Autodesk Fusion 360 part; units mm, degrees
note: some values were not read from the file. Set by a fixed rule: which sketch regions a step uses.
(part 14 of 20)
  spline S78 degree 5 poles (15.0758, 27.0873) (15.0737, 27.0855) (15.0696, 27.082) (15.0635, 27.0767) (15.0553, 27.0697) (15.045, 27.061) (15.0349, 27.0522) (15.0247, 27.0435) (15.0146, 27.0347) (15.0045, 27.026) (14.9945, 27.0173) (14.9845, 27.0086) (14.9745, 26.9999) (14.9646, 26.9912) (14.9547, 26.9825) (14.9448, 26.9738) (14.935, 26.9651) (14.9252, 26.9565) (14.9154, 26.9478) (14.9057, 26.9392) (14.896, 26.9305) (14.8863, 26.9219) (14.8767, 26.9133) (14.8671, 26.9047) (14.8576, 26.8961) (14.8481, 26.8875) (14.8386, 26.8789) (14.8291, 26.8703) (14.8197, 26.8618) (14.8104, 26.8532) (14.801, 26.8447) (14.7917, 26.8361) (14.7824, 26.8276) (14.7732, 26.8191) (14.764, 26.8106) (14.7549, 26.8021) (14.7457, 26.7937) (14.7366, 26.7852) (14.7276, 26.7767) (14.7186, 26.7683) (14.7096, 26.7599) (14.7006, 26.7515) (14.6917, 26.7431) (14.6829, 26.7347) (14.674, 26.7263) (14.6652, 26.7179) (14.6565, 26.7096) (14.6477, 26.7012) (14.639, 26.6929) (14.6304, 26.6846) (14.6218, 26.6763) (14.6132, 26.668) (14.6046, 26.6597) (14.5961, 26.6514) (14.5877, 26.6432) (14.5792, 26.635) (14.5708, 26.6267) (14.5625, 26.6185) (14.5541, 26.6103) (14.5459, 26.6022) (14.5376, 26.594) (14.5294, 26.5858) (14.5212, 26.5777) (14.5131, 26.5696) (14.505, 26.5615) (14.4969, 26.5534) (14.4889, 26.5453) (14.4809, 26.5373) (14.4729, 26.5292) (14.465, 26.5212) (14.4571, 26.5132) (14.4493, 26.5052) (14.4415, 26.4972) (14.4337, 26.4893) (14.426, 26.4813) (14.4183, 26.4734) (14.4106, 26.4655) (14.403, 26.4576) (14.3954, 26.4497) (14.3879, 26.4419) (14.3804, 26.434) (14.3729, 26.4262) (14.3655, 26.4184) (14.3581, 26.4106) (14.3508, 26.4029) (14.3435, 26.3951) (14.3362, 26.3874) (14.3289, 26.3797) (14.3217, 26.372) (14.3146, 26.3643) (14.3075, 26.3567) (14.3004, 26.3491) (14.2933, 26.3414) (14.2863, 26.3339) (14.2794, 26.3263) (14.2724, 26.3188) (14.2656, 26.3112) (14.2587, 26.3037) (14.2519, 26.2962) (14.2451, 26.2888) (14.2384, 26.2813) (14.2317, 26.2739) (14.225, 26.2665) (14.2184, 26.2592) (14.2119, 26.2518) (14.2053, 26.2445) (14.1988, 26.2372) (14.1924, 26.2299) (14.1859, 26.2227) (14.1796, 26.2154) (14.1732, 26.2082) (14.1669, 26.201) (14.1607, 26.1939) (14.1544, 26.1868) (14.1483, 26.1796) (14.1421, 26.1726) (14.136, 26.1655) (14.13, 26.1585) (14.1239, 26.1515) (14.118, 26.1445) (14.112, 26.1375) (14.1061, 26.1306) (14.1003, 26.1237) (14.0945, 26.1168) (14.0887, 26.11) (14.0829, 26.1032) (14.0772, 26.0964) (14.0716, 26.0896) (14.066, 26.0829) (14.0604, 26.0762) (14.0549, 26.0695) (14.0494, 26.0629) (14.0439, 26.0563) (14.0385, 26.0497) (14.0332, 26.0431) (14.0278, 26.0366) (14.0225, 26.0301) (14.0173, 26.0236) (14.0121, 26.0172) (14.0069, 26.0108) (14.0018, 26.0044) (13.9967, 25.9981) (13.9917, 25.9918) (13.9867, 25.9855) (13.9818, 25.9793) (13.9769, 25.9731) (13.972, 25.9669) (13.9672, 25.9608) (13.9624, 25.9547) (13.9576, 25.9486) (13.9529, 25.9426) (13.9483, 25.9366) (13.9437, 25.9306) (13.9391, 25.9247) (13.9346, 25.9188) (13.9301, 25.913) (13.9257, 25.9072) (13.9213, 25.9014) (13.9169, 25.8957) (13.9126, 25.89) (13.9083, 25.8843) (13.9041, 25.8787) (13.8999, 25.8731) (13.8958, 25.8676) (13.8917, 25.8621) (13.8876, 25.8566) (13.8836, 25.8512) (13.8797, 25.8458) (13.8758, 25.8405) (13.8719, 25.8352) (13.8681, 25.8299) (13.8643, 25.8247) (13.8605, 25.8195) (13.8568, 25.8144) (13.8532, 25.8093) (13.8496, 25.8043) (13.846, 25.7993) (13.8425, 25.7944) (13.839, 25.7895) (13.8356, 25.7847) (13.8322, 25.7799) (13.8289, 25.7751) (13.8256, 25.7704) (13.8224, 25.7658) (13.8192, 25.7612) (13.816, 25.7566) (13.8129, 25.7521) (13.8098, 25.7476) (13.8068, 25.7432) (13.8039, 25.7389) (13.8009, 25.7346) (13.7981, 25.7304) (13.7952, 25.7262) (13.7925, 25.722) (13.7897, 25.718) (13.787, 25.7139) (13.7844, 25.71) (13.7818, 25.706) (13.7793, 25.7022) (13.7768, 25.6984) (13.7743, 25.6947) (13.7719, 25.691) (13.7696, 25.6874) (13.7673, 25.6838) (13.765, 25.6803) (13.7628, 25.6769) (13.7607, 25.6735) (13.7586, 25.6702) (13.7565, 25.667) (13.7545, 25.6638) (13.7526, 25.6607) (13.7506, 25.6577) (13.7488, 25.6547) (13.747, 25.6518) (13.7452, 25.6489) (13.7435, 25.6462) (13.7419, 25.6435) (13.7403, 25.6409) (13.7387, 25.6383) (13.7372, 25.6358) (13.7358, 25.6334) (13.7344, 25.6311) (13.733, 25.6289) (13.7317, 25.6267) (13.7305, 25.6246) (13.7293, 25.6226) (13.7282, 25.6207) (13.7271, 25.6188) (13.7261, 25.6171) (13.7251, 25.6154) (13.7242, 25.6138) (13.7233, 25.6123) (13.7225, 25.6109) (13.7217, 25.6096) (13.721, 25.6083) (13.7204, 25.6072) (13.7198, 25.6061) (13.7193, 25.6052) (13.7188, 25.6043) (13.7184, 25.6036) (13.718, 25.6029) (13.7178, 25.6025) (13.7176, 25.6022) (13.7175, 25.602) (13.7175, 25.6019) knots -1 -1 -1 -1 -1 -1 -0.99583333 -0.99166667 -0.9875 -0.98333333 -0.97916667 -0.975 -0.97083333 -0.96666667 -0.9625 -0.95833333 -0.95416667 -0.95 -0.94583333 -0.94166667 -0.9375 -0.93333333 -0.92916667 -0.925 -0.92083333 -0.91666667 -0.9125 -0.90833333 -0.90416667 -0.9 -0.89583333 -0.89166667 -0.8875 -0.88333333 -0.87916667 -0.875 -0.87083333 -0.86666667 -0.8625 -0.85833333 -0.85416667 -0.85 -0.84583333 -0.84166667 -0.8375 -0.83333333 -0.82916667 -0.825 -0.82083333 -0.81666667 -0.8125 -0.80833333 -0.80416667 -0.8 -0.79583333 -0.79166667 -0.7875 -0.78333333 -0.77916667 -0.775 -0.77083333 -0.76666667 -0.7625 -0.75833333 -0.75416667 -0.75 -0.74583333 -0.74166667 -0.7375 -0.73333333 -0.72916667 -0.725 -0.72083333 -0.71666667 -0.7125 -0.70833333 -0.70416667 -0.7 -0.69583333 -0.69166667 -0.6875 -0.68333333 -0.67916667 -0.675 -0.67083333 -0.66666667 -0.6625 -0.65833333 -0.65416667 -0.65 -0.64583333 -0.64166667 -0.6375 -0.63333333 -0.62916667 -0.625 -0.62083333 -0.61666667 -0.6125 -0.60833333 -0.60416667 -0.6 -0.59583333 -0.59166667 -0.5875 -0.58333333 -0.57916667 -0.575 -0.57083333 -0.56666667 -0.5625 -0.55833333 -0.55416667 -0.55 -0.54583333 -0.54166667 -0.5375 -0.53333333 -0.52916667 -0.525 -0.52083333 -0.51666667 -0.5125 -0.50833333 -0.50416667 -0.5 -0.49583333 -0.49166667 -0.4875 -0.48333333 -0.47916667 -0.475 -0.47083333 -0.46666667 -0.4625 -0.45833333 -0.45416667 -0.45 -0.44583333 -0.44166667 -0.4375 -0.43333333 -0.42916667 -0.425 -0.42083333 -0.41666667 -0.4125 -0.40833333 -0.40416667 -0.4 -0.39583333 -0.39166667 -0.3875 -0.38333333 -0.37916667 -0.375 -0.37083333 -0.36666667 -0.3625 -0.35833333 -0.35416667 -0.35 -0.34583333 -0.34166667 -0.3375 -0.33333333 -0.32916667 -0.325 -0.32083333 -0.31666667 -0.3125 -0.30833333 -0.30416667 -0.3 -0.29583333 -0.29166667 -0.2875 -0.28333333 -0.27916667 -0.275 -0.27083333 -0.26666667 -0.2625 -0.25833333 -0.25416667 -0.25 -0.24583333 -0.24166667 -0.2375 -0.23333333 -0.22916667 -0.225 -0.22083333 -0.21666667 -0.2125 -0.20833333 -0.20416667 -0.2 -0.19583333 -0.19166667 -0.1875 -0.18333333 -0.17916667 -0.175 -0.17083333 -0.16666667 -0.1625 -0.15833333 -0.15416667 -0.15 -0.14583333 -0.14166667 -0.1375 -0.13333333 -0.12916667 -0.125 -0.12083333 -0.11666667 -0.1125 -0.10833333 -0.10416667 -0.1 -0.09583333 -0.09166667 -0.0875 -0.08333333 -0.07916667 -0.075 -0.07083333 -0.06666667 -0.0625 -0.05833333 -0.05416667 -0.05 -0.04583333 -0.04166667 -0.0375 -0.03333333 -0.02916667 -0.025 -0.02083333 -0.01666667 -0.0125 -0.00833333 -0.00416667 0 0 0 0 0 0
  line L164 (-13.578, 25.3417) -> (-13.7171, 25.6012)
  line L165 (-12.6495, 26.1461) -> (-12.6491, 26.1453)
  spline S79 degree 5 poles (17.8246, 25.363) (17.8224, 25.3615) (17.8179, 25.3584) (17.8112, 25.3539) (17.8023, 25.3477) (17.7913, 25.3401) (17.7802, 25.3325) (17.7692, 25.3248) (17.7583, 25.3172) (17.7473, 25.3096) (17.7364, 25.3019) (17.7256, 25.2943) (17.7147, 25.2867) (17.7039, 25.2791) (17.6932, 25.2715) (17.6825, 25.2639) (17.6718, 25.2563) (17.6611, 25.2487) (17.6505, 25.2411) (17.6399, 25.2335) (17.6294, 25.2259) (17.6189, 25.2184) (17.6084, 25.2108) (17.598, 25.2032) (17.5876, 25.1957) (17.5772, 25.1881) (17.5669, 25.1806) (17.5566, 25.1731) (17.5464, 25.1655) (17.5361, 25.158) (17.526, 25.1505) (17.5158, 25.143) (17.5057, 25.1355) (17.4956, 25.128) (17.4856, 25.1205) (17.4756, 25.113) (17.4657, 25.1055) (17.4557, 25.0981) (17.4458, 25.0906) (17.436, 25.0832) (17.4262, 25.0757) (17.4164, 25.0683) (17.4067, 25.0609) (17.397, 25.0534) (17.3873, 25.046) (17.3777, 25.0386) (17.3681, 25.0312) (17.3585, 25.0238) (17.349, 25.0165) (17.3395, 25.0091) (17.3301, 25.0017) (17.3207, 24.9944) (17.3113, 24.9871) (17.302, 24.9797) (17.2927, 24.9724) (17.2835, 24.9651) (17.2743, 24.9578) (17.2651, 24.9505) (17.2559, 24.9432) (17.2469, 24.936) (17.2378, 24.9287) (17.2288, 24.9215) (17.2198, 24.9142) (17.2108, 24.907) (17.2019, 24.8998) (17.1931, 24.8926) (17.1842, 24.8854) (17.1754, 24.8782) (17.1667, 24.8711) (17.158, 24.8639) (17.1493, 24.8568) (17.1407, 24.8496) (17.1321, 24.8425) (17.1235, 24.8354) (17.115, 24.8283) (17.1065, 24.8212) (17.0981, 24.8142) (17.0897, 24.8071) (17.0813, 24.8001) (17.073, 24.7931) (17.0647, 24.7861) (17.0565, 24.7791) (17.0483, 24.7721) (17.0401, 24.7651) (17.032, 24.7582) (17.0239, 24.7512) (17.0159, 24.7443) (17.0079, 24.7374) (16.9999, 24.7305) (16.992, 24.7236) (16.9841, 24.7168) (16.9763, 24.7099) (16.9685, 24.7031) (16.9607, 24.6963) (16.953, 24.6895) (16.9453, 24.6827) (16.9377, 24.6759) (16.9301, 24.6692) (16.9225, 24.6625) (16.915, 24.6558) (16.9075, 24.6491) (16.9001, 24.6424) (16.8927, 24.6357) (16.8854, 24.6291) (16.8781, 24.6225) (16.8708, 24.6159) (16.8636, 24.6093) (16.8564, 24.6027) (16.8492, 24.5962) (16.8421, 24.5897) (16.8351, 24.5831) (16.8281, 24.5767) (16.8211, 24.5702) (16.8142, 24.5638) (16.8073, 24.5573) (16.8004, 24.5509) (16.7936, 24.5446) (16.7869, 24.5382) (16.7801, 24.5319) (16.7735, 24.5255) (16.7668, 24.5192) (16.7602, 24.513) (16.7537, 24.5067) (16.7472, 24.5005) (16.7407, 24.4943) (16.7343, 24.4881) (16.7279, 24.482) (16.7216, 24.4758) (16.7153, 24.4697) (16.7091, 24.4636) (16.7029, 24.4576) (16.6967, 24.4515) (16.6906, 24.4455) (16.6845, 24.4395) (16.6785, 24.4336) (16.6725, 24.4277) (16.6666, 24.4218) (16.6607, 24.4159) (16.6549, 24.41) (16.6491, 24.4042) (16.6433, 24.3984) (16.6376, 24.3926) (16.6319, 24.3869) (16.6263, 24.3812) (16.6207, 24.3755) (16.6152, 24.3698) (16.6097, 24.3642) (16.6043, 24.3586) (16.5989, 24.353) (16.5935, 24.3475) (16.5882, 24.342) (16.583, 24.3365) (16.5778, 24.3311) (16.5726, 24.3257) (16.5675, 24.3203) (16.5624, 24.3149) (16.5574, 24.3096) (16.5524, 24.3043) (16.5475, 24.2991) (16.5426, 24.2939) (16.5378, 24.2887) (16.533, 24.2835) (16.5282, 24.2784) (16.5236, 24.2733) (16.5189, 24.2683) (16.5143, 24.2633) (16.5098, 24.2583) (16.5053, 24.2534) (16.5008, 24.2485) (16.4964, 24.2436) (16.492, 24.2388) (16.4877, 24.234) (16.4835, 24.2293) (16.4793, 24.2246) (16.4751, 24.2199) (16.471, 24.2153) (16.4669, 24.2107) (16.4629, 24.2062) (16.459, 24.2017) (16.455, 24.1972) (16.4512, 24.1928) (16.4474, 24.1884) (16.4436, 24.1841) (16.4399, 24.1798) (16.4362, 24.1755) (16.4326, 24.1713) (16.4291, 24.1672) (16.4256, 24.1631) (16.4221, 24.159) (16.4187, 24.155) (16.4153, 24.151) (16.412, 24.1471) (16.4088, 24.1432) (16.4056, 24.1394) (16.4024, 24.1356) (16.3994, 24.1319) (16.3963, 24.1283) (16.3933, 24.1246) (16.3904, 24.1211) (16.3875, 24.1176) (16.3847, 24.1141) (16.3819, 24.1107) (16.3792, 24.1073) (16.3766, 24.104) (16.374, 24.1008) (16.3714, 24.0976) (16.3689, 24.0945) (16.3665, 24.0914) (16.3641, 24.0884) (16.3618, 24.0855) (16.3595, 24.0826) (16.3573, 24.0798) (16.3551, 24.077) (16.353, 24.0743) (16.351, 24.0717) (16.349, 24.0691) (16.3471, 24.0666) (16.3452, 24.0641) (16.3434, 24.0618) (16.3416, 24.0595) (16.3399, 24.0572) (16.3383, 24.0551) (16.3367, 24.053) (16.3352, 24.051) (16.3338, 24.049) (16.3324, 24.0471) (16.331, 24.0453) (16.3298, 24.0436) (16.3286, 24.042) (16.3274, 24.0404) (16.3263, 24.0389) (16.3253, 24.0375) (16.3244, 24.0362) (16.3235, 24.035) (16.3227, 24.0338) (16.3219, 24.0327) (16.3212, 24.0317) (16.3206, 24.0309) (16.32, 24.0301) (16.3195, 24.0294) (16.3191, 24.0287) (16.3188, 24.0283) (16.3186, 24.0281) (16.3185, 24.0279) (16.3184, 24.0278) knots -1 -1 -1 -1 -1 -1 -0.99583333 -0.99166667 -0.9875 -0.98333333 -0.97916667 -0.975 -0.97083333 -0.96666667 -0.9625 -0.95833333 -0.95416667 -0.95 -0.94583333 -0.94166667 -0.9375 -0.93333333 -0.92916667 -0.925 -0.92083333 -0.91666667 -0.9125 -0.90833333 -0.90416667 -0.9 -0.89583333 -0.89166667 -0.8875 -0.88333333 -0.87916667 -0.875 -0.87083333 -0.86666667 -0.8625 -0.85833333 -0.85416667 -0.85 -0.84583333 -0.84166667 -0.8375 -0.83333333 -0.82916667 -0.825 -0.82083333 -0.81666667 -0.8125 -0.80833333 -0.80416667 -0.8 -0.79583333 -0.79166667 -0.7875 -0.78333333 -0.77916667 -0.775 -0.77083333 -0.76666667 -0.7625 -0.75833333 -0.75416667 -0.75 -0.74583333 -0.74166667 -0.7375 -0.73333333 -0.72916667 -0.725 -0.72083333 -0.71666667 -0.7125 -0.70833333 -0.70416667 -0.7 -0.69583333 -0.69166667 -0.6875 -0.68333333 -0.67916667 -0.675 -0.67083333 -0.66666667 -0.6625 -0.65833333 -0.65416667 -0.65 -0.64583333 -0.64166667 -0.6375 -0.63333333 -0.62916667 -0.625 -0.62083333 -0.61666667 -0.6125 -0.60833333 -0.60416667 -0.6 -0.59583333 -0.59166667 -0.5875 -0.58333333 -0.57916667 -0.575 -0.57083333 -0.56666667 -0.5625 -0.55833333 -0.55416667 -0.55 -0.54583333 -0.54166667 -0.5375 -0.53333333 -0.52916667 -0.525 -0.52083333 -0.51666667 -0.5125 -0.50833333 -0.50416667 -0.5 -0.49583333 -0.49166667 -0.4875 -0.48333333 -0.47916667 -0.475 -0.47083333 -0.46666667 -0.4625 -0.45833333 -0.45416667 -0.45 -0.44583333 -0.44166667 -0.4375 -0.43333333 -0.42916667 -0.425 -0.42083333 -0.41666667 -0.4125 -0.40833333 -0.40416667 -0.4 -0.39583333 -0.39166667 -0.3875 -0.38333333 -0.37916667 -0.375 -0.37083333 -0.36666667 -0.3625 -0.35833333 -0.35416667 -0.35 -0.34583333 -0.34166667 -0.3375 -0.33333333 -0.32916667 -0.325 -0.32083333 -0.31666667 -0.3125 -0.30833333 -0.30416667 -0.3 -0.29583333 -0.29166667 -0.2875 -0.28333333 -0.27916667 -0.275 -0.27083333 -0.26666667 -0.2625 -0.25833333 -0.25416667 -0.25 -0.24583333 -0.24166667 -0.2375 -0.23333333 -0.22916667 -0.225 -0.22083333 -0.21666667 -0.2125 -0.20833333 -0.20416667 -0.2 -0.19583333 -0.19166667 -0.1875 -0.18333333 -0.17916667 -0.175 -0.17083333 -0.16666667 -0.1625 -0.15833333 -0.15416667 -0.15 -0.14583333 -0.14166667 -0.1375 -0.13333333 -0.12916667 -0.125 -0.12083333 -0.11666667 -0.1125 -0.10833333 -0.10416667 -0.1 -0.09583333 -0.09166667 -0.0875 -0.08333333 -0.07916667 -0.075 -0.07083333 -0.06666667 -0.0625 -0.05833333 -0.05416667 -0.05 -0.04583333 -0.04166667 -0.0375 -0.03333333 -0.02916667 -0.025 -0.02083333 -0.01666667 -0.0125 -0.00833333 -0.00416667 0 0 0 0 0 0
  arc A80 (15.9204, 26.5997) -> (15.0758, 27.0873) centre (0, 0) ccw
  arc A81 (16.1526, 23.7836) -> (15.1575, 24.4297) centre (0, 0) ccw
  line L166 (-10.9659, 26.8948) -> (-10.9662, 26.8955)
  line L167 (12.5209, 25.8803) -> (12.6491, 26.1453)
  line L168 (-8.0948, -27.8945) -> (-8.0945, -27.8937)
  line L169 (-13.7171, 25.6012) -> (-13.7175, 25.6019)
  spline S80 degree 5 poles (-10.0421, 29.3284) (-10.0422, 29.3257) (-10.0423, 29.3203) (-10.0425, 29.3122) (-10.0428, 29.3014) (-10.0431, 29.288) (-10.0434, 29.2745) (-10.0437, 29.2612) (-10.044, 29.2478) (-10.0442, 29.2345) (-10.0445, 29.2212) (-10.0447, 29.2079) (-10.0449, 29.1947) (-10.0451, 29.1815) (-10.0453, 29.1683) (-10.0454, 29.1551) (-10.0455, 29.142) (-10.0457, 29.129) (-10.0458, 29.1159) (-10.0458, 29.1029) (-10.0459, 29.0899) (-10.046, 29.077) (-10.046, 29.0641) (-10.046, 29.0512) (-10.046, 29.0383) (-10.046, 29.0255) (-10.046, 29.0127) (-10.0459, 29) (-10.0458, 28.9872) (-10.0458, 28.9745) (-10.0457, 28.9619) (-10.0456, 28.9493) (-10.0454, 28.9367) (-10.0453, 28.9241) (-10.0451, 28.9116) (-10.0449, 28.8991) (-10.0448, 28.8867) (-10.0445, 28.8743) (-10.0443, 28.8619) (-10.0441, 28.8495) (-10.0438, 28.8372) (-10.0436, 28.8249) (-10.0433, 28.8127) (-10.043, 28.8005) (-10.0427, 28.7883) (-10.0423, 28.7762) (-10.042, 28.7641) (-10.0416, 28.752) (-10.0412, 28.74) (-10.0409, 28.728) (-10.0405, 28.716) (-10.04, 28.7041) (-10.0396, 28.6922) (-10.0392, 28.6803) (-10.0387, 28.6685) (-10.0382, 28.6567) (-10.0377, 28.645) (-10.0372, 28.6333) (-10.0367, 28.6216) (-10.0362, 28.61) (-10.0356, 28.5984) (-10.0351, 28.5868) (-10.0345, 28.5753) (-10.0339, 28.5638) (-10.0333, 28.5524) (-10.0327, 28.541) (-10.0321, 28.5296) (-10.0314, 28.5183) (-10.0308, 28.507) (-10.0301, 28.4957) (-10.0294, 28.4845) (-10.0287, 28.4733) (-10.028, 28.4622) (-10.0273, 28.4511) (-10.0266, 28.44) (-10.0258, 28.429) (-10.0251, 28.4181) (-10.0243, 28.4071) (-10.0235, 28.3962) (-10.0227, 28.3854) (-10.0219, 28.3745) (-10.0211, 28.3638) (-10.0203, 28.353) (-10.0195, 28.3423) (-10.0186, 28.3317) (-10.0177, 28.321) (-10.0169, 28.3105) (-10.016, 28.2999) (-10.0151, 28.2894) (-10.0142, 28.279) (-10.0133, 28.2686) (-10.0123, 28.2582) (-10.0114, 28.2479) (-10.0104, 28.2376) (-10.0095, 28.2274) (-10.0085, 28.2172) (-10.0075, 28.207) (-10.0065, 28.1969) (-10.0055, 28.1868) (-10.0045, 28.1768) (-10.0035, 28.1668) (-10.0025, 28.1569) (-10.0014, 28.147) (-10.0004, 28.1372) (-9.9993, 28.1274) (-9.9983, 28.1176) (-9.9972, 28.1079) (-9.9961, 28.0982) (-9.995, 28.0886) (-9.9939, 28.079) (-9.9928, 28.0695) (-9.9916, 28.06) (-9.9905, 28.0506) (-9.9894, 28.0412) (-9.9882, 28.0318) (-9.9871, 28.0225) (-9.9859, 28.0133) (-9.9847, 28.004) (-9.9836, 27.9949) (-9.9824, 27.9858) (-9.9812, 27.9767) (-9.98, 27.9677) (-9.9788, 27.9587) (-9.9776, 27.9498) (-9.9763, 27.9409) (-9.9751, 27.9321) (-9.9739, 27.9233) (-9.9726, 27.9146) (-9.9714, 27.9059) (-9.9701, 27.8973) (-9.9689, 27.8887) (-9.9676, 27.8802) (-9.9664, 27.8717) (-9.9651, 27.8633) (-9.9638, 27.8549) (-9.9625, 27.8466) (-9.9612, 27.8383) (-9.9599, 27.8301) (-9.9586, 27.8219) (-9.9573, 27.8138) (-9.956, 27.8057) (-9.9547, 27.7977) (-9.9534, 27.7898) (-9.9521, 27.7819) (-9.9508, 27.774) (-9.9494, 27.7662) (-9.9481, 27.7585) (-9.9468, 27.7508) (-9.9454, 27.7431) (-9.9441, 27.7356) (-9.9428, 27.728) (-9.9414, 27.7206) (-9.9401, 27.7132) (-9.9387, 27.7058) (-9.9374, 27.6985) (-9.936, 27.6912) (-9.9347, 27.6841) (-9.9333, 27.6769) (-9.932, 27.6698) (-9.9306, 27.6628) (-9.9293, 27.6559) (-9.9279, 27.649) (-9.9266, 27.6421) (-9.9252, 27.6353) (-9.9239, 27.6286) (-9.9225, 27.622) (-9.9212, 27.6154) (-9.9199, 27.6088) (-9.9185, 27.6023) (-9.9172, 27.5959) (-9.9158, 27.5896) (-9.9145, 27.5833) (-9.9132, 27.577) (-9.9118, 27.5709) (-9.9105, 27.5647) (-9.9092, 27.5587) (-9.9079, 27.5527) (-9.9065, 27.5468) (-9.9052, 27.5409) (-9.9039, 27.5352) (-9.9026, 27.5294) (-9.9013, 27.5238) (-9.9, 27.5182) (-9.8987, 27.5127) (-9.8974, 27.5072) (-9.8962, 27.5018) (-9.8949, 27.4965) (-9.8936, 27.4912) (-9.8924, 27.4861) (-9.8911, 27.481) (-9.8899, 27.4759) (-9.8887, 27.4709) (-9.8874, 27.466) (-9.8862, 27.4612) (-9.885, 27.4564) (-9.8838, 27.4517) (-9.8827, 27.4471) (-9.8815, 27.4426) (-9.8803, 27.4381) (-9.8792, 27.4337) (-9.878, 27.4294) (-9.8769, 27.4252) (-9.8758, 27.421) (-9.8747, 27.4169) (-9.8736, 27.4129) (-9.8725, 27.409) (-9.8715, 27.4051) (-9.8704, 27.4013) (-9.8694, 27.3976) (-9.8684, 27.394) (-9.8674, 27.3905) (-9.8664, 27.387) (-9.8654, 27.3837) (-9.8645, 27.3804) (-9.8635, 27.3772) (-9.8626, 27.3741) (-9.8617, 27.371) (-9.8608, 27.3681) (-9.86, 27.3652) (-9.8591, 27.3625) (-9.8583, 27.3598) (-9.8575, 27.3572) (-9.8568, 27.3547) (-9.856, 27.3523) (-9.8553, 27.3499) (-9.8546, 27.3477) (-9.8539, 27.3456) (-9.8533, 27.3435) (-9.8527, 27.3416) (-9.8521, 27.3398) (-9.8515, 27.338) (-9.851, 27.3364) (-9.8505, 27.3348) (-9.85, 27.3334) (-9.8495, 27.332) (-9.8491, 27.3308) (-9.8487, 27.3296) (-9.8484, 27.3286) (-9.8481, 27.3277) (-9.8478, 27.3269) (-9.8475, 27.3262) (-9.8474, 27.3257) (-9.8473, 27.3254) (-9.8472, 27.3252) (-9.8472, 27.3251) knots -1 -1 -1 -1 -1 -1 -0.99583333 -0.99166667 -0.9875 -0.98333333 -0.97916667 -0.975 -0.97083333 -0.96666667 -0.9625 -0.95833333 -0.95416667 -0.95 -0.94583333 -0.94166667 -0.9375 -0.93333333 -0.92916667 -0.925 -0.92083333 -0.91666667 -0.9125 -0.90833333 -0.90416667 -0.9 -0.89583333 -0.89166667 -0.8875 -0.88333333 -0.87916667 -0.875 -0.87083333 -0.86666667 -0.8625 -0.85833333 -0.85416667 -0.85 -0.84583333 -0.84166667 -0.8375 -0.83333333 -0.82916667 -0.825 -0.82083333 -0.81666667 -0.8125 -0.80833333 -0.80416667 -0.8 -0.79583333 -0.79166667 -0.7875 -0.78333333 -0.77916667 -0.775 -0.77083333 -0.76666667 -0.7625 -0.75833333 -0.75416667 -0.75 -0.74583333 -0.74166667 -0.7375 -0.73333333 -0.72916667 -0.725 -0.72083333 -0.71666667 -0.7125 -0.70833333 -0.70416667 -0.7 -0.69583333 -0.69166667 -0.6875 -0.68333333 -0.67916667 -0.675 -0.67083333 -0.66666667 -0.6625 -0.65833333 -0.65416667 -0.65 -0.64583333 -0.64166667 -0.6375 -0.63333333 -0.62916667 -0.625 -0.62083333 -0.61666667 -0.6125 -0.60833333 -0.60416667 -0.6 -0.59583333 -0.59166667 -0.5875 -0.58333333 -0.57916667 -0.575 -0.57083333 -0.56666667 -0.5625 -0.55833333 -0.55416667 -0.55 -0.54583333 -0.54166667 -0.5375 -0.53333333 -0.52916667 -0.525 -0.52083333 -0.51666667 -0.5125 -0.50833333 -0.50416667 -0.5 -0.49583333 -0.49166667 -0.4875 -0.48333333 -0.47916667 -0.475 -0.47083333 -0.46666667 -0.4625 -0.45833333 -0.45416667 -0.45 -0.44583333 -0.44166667 -0.4375 -0.43333333 -0.42916667 -0.425 -0.42083333 -0.41666667 -0.4125 -0.40833333 -0.40416667 -0.4 -0.39583333 -0.39166667 -0.3875 -0.38333333 -0.37916667 -0.375 -0.37083333 -0.36666667 -0.3625 -0.35833333 -0.35416667 -0.35 -0.34583333 -0.34166667 -0.3375 -0.33333333 -0.32916667 -0.325 -0.32083333 -0.31666667 -0.3125 -0.30833333 -0.30416667 -0.3 -0.29583333 -0.29166667 -0.2875 -0.28333333 -0.27916667 -0.275 -0.27083333 -0.26666667 -0.2625 -0.25833333 -0.25416667 -0.25 -0.24583333 -0.24166667 -0.2375 -0.23333333 -0.22916667 -0.225 -0.22083333 -0.21666667 -0.2125 -0.20833333 -0.20416667 -0.2 -0.19583333 -0.19166667 -0.1875 -0.18333333 -0.17916667 -0.175 -0.17083333 -0.16666667 -0.1625 -0.15833333 -0.15416667 -0.15 -0.14583333 -0.14166667 -0.1375 -0.13333333 -0.12916667 -0.125 -0.12083333 -0.11666667 -0.1125 -0.10833333 -0.10416667 -0.1 -0.09583333 -0.09166667 -0.0875 -0.08333333 -0.07916667 -0.075 -0.07083333 -0.06666667 -0.0625 -0.05833333 -0.05416667 -0.05 -0.04583333 -0.04166667 -0.0375 -0.03333333 -0.02916667 -0.025 -0.02083333 -0.01666667 -0.0125 -0.00833333 -0.00416667 0 0 0 0 0 0
  line L170 (13.7171, 25.6012) -> (13.578, 25.3417)
  spline S81 degree 5 poles (-10.9662, 26.8955) (-10.9662, 26.8956) (-10.9663, 26.8958) (-10.9664, 26.8961) (-10.9666, 26.8966) (-10.9669, 26.8973) (-10.9672, 26.8981) (-10.9676, 26.899) (-10.9681, 26.9) (-10.9685, 26.9011) (-10.9691, 26.9023) (-10.9696, 26.9036) (-10.9702, 26.905) (-10.9709, 26.9065) (-10.9716, 26.908) (-10.9724, 26.9097) (-10.9731, 26.9115) (-10.974, 26.9134) (-10.9749, 26.9153) (-10.9758, 26.9173) (-10.9768, 26.9195) (-10.9778, 26.9217) (-10.9788, 26.924) (-10.9799, 26.9263) (-10.9811, 26.9288) (-10.9823, 26.9313) (-10.9835, 26.9339) (-10.9848, 26.9366) (-10.9861, 26.9394) (-10.9875, 26.9423) (-10.9889, 26.9452) (-10.9903, 26.9482) (-10.9918, 26.9513) (-10.9934, 26.9544) (-10.9949, 26.9577) (-10.9966, 26.961) (-10.9982, 26.9643) (-10.9999, 26.9678) (-11.0017, 26.9713) (-11.0035, 26.9748) (-11.0053, 26.9785) (-11.0072, 26.9822) (-11.0091, 26.986) (-11.0111, 26.9898) (-11.0131, 26.9937) (-11.0151, 26.9977) (-11.0172, 27.0017) (-11.0193, 27.0058) (-11.0215, 27.01) (-11.0237, 27.0142) (-11.0259, 27.0185) (-11.0282, 27.0228) (-11.0306, 27.0272) (-11.0329, 27.0317) (-11.0353, 27.0362) (-11.0378, 27.0408) (-11.0403, 27.0454) (-11.0428, 27.0501) (-11.0454, 27.0549) (-11.048, 27.0597) (-11.0507, 27.0645) (-11.0534, 27.0694) (-11.0561, 27.0744) (-11.0589, 27.0794) (-11.0617, 27.0845) (-11.0646, 27.0896) (-11.0675, 27.0948) (-11.0704, 27.1) (-11.0734, 27.1053) (-11.0764, 27.1106) (-11.0795, 27.116) (-11.0826, 27.1214) (-11.0857, 27.1269) (-11.0889, 27.1324) (-11.0921, 27.138) (-11.0954, 27.1436) (-11.0987, 27.1493) (-11.102, 27.155) (-11.1054, 27.1608) (-11.1088, 27.1666) (-11.1123, 27.1725) (-11.1158, 27.1784) (-11.1193, 27.1843) (-11.1229, 27.1903) (-11.1265, 27.1963) (-11.1301, 27.2024) (-11.1338, 27.2085) (-11.1376, 27.2147) (-11.1413, 27.2209) (-11.1451, 27.2271) (-11.149, 27.2334) (-11.1529, 27.2397) (-11.1568, 27.2461) (-11.1608, 27.2525) (-11.1648, 27.259) (-11.1688, 27.2654) (-11.1729, 27.272) (-11.177, 27.2785) (-11.1812, 27.2851) (-11.1854, 27.2918) (-11.1896, 27.2985) (-11.1939, 27.3052) (-11.1982, 27.3119) (-11.2025, 27.3187) (-11.2069, 27.3256) (-11.2113, 27.3324) (-11.2158, 27.3393) (-11.2203, 27.3463) (-11.2248, 27.3533) (-11.2294, 27.3603) (-11.234, 27.3673) (-11.2387, 27.3744) (-11.2434, 27.3815) (-11.2481, 27.3887) (-11.2529, 27.3958) (-11.2577, 27.4031) (-11.2625, 27.4103) (-11.2674, 27.4176) (-11.2723, 27.4249) (-11.2773, 27.4323) (-11.2823, 27.4396) (-11.2873, 27.447) (-11.2924, 27.4545) (-11.2975, 27.462) (-11.3026, 27.4695) (-11.3078, 27.477) (-11.313, 27.4846) (-11.3183, 27.4922) (-11.3235, 27.4998) (-11.3289, 27.5074) (-11.3342, 27.5151) (-11.3396, 27.5228) (-11.3451, 27.5306) (-11.3506, 27.5384) (-11.3561, 27.5462) (-11.3616, 27.554) (-11.3672, 27.5618) (-11.3728, 27.5697) (-11.3785, 27.5776) (-11.3842, 27.5856) (-11.3899, 27.5936) (-11.3957, 27.6015) (-11.4015, 27.6096) (-11.4074, 27.6176) (-11.4132, 27.6257) (-11.4192, 27.6338) (-11.4251, 27.6419) (-11.4311, 27.6501) (-11.4371, 27.6582) (-11.4432, 27.6665) (-11.4493, 27.6747) (-11.4554, 27.6829) (-11.4616, 27.6912) (-11.4678, 27.6995) (-11.4741, 27.7078) (-11.4803, 27.7162) (-11.4867, 27.7246) (-11.493, 27.733) (-11.4994, 27.7414) (-11.5058, 27.7498) (-11.5123, 27.7583) (-11.5188, 27.7668) (-11.5253, 27.7753) (-11.5319, 27.7838) (-11.5385, 27.7924) (-11.5452, 27.801) (-11.5518, 27.8096) (-11.5585, 27.8182) (-11.5653, 27.8268) (-11.5721, 27.8355) (-11.5789, 27.8442) (-11.5858, 27.8529) (-11.5927, 27.8616) (-11.5996, 27.8704) (-11.6065, 27.8791) (-11.6135, 27.8879) (-11.6206, 27.8967) (-11.6276, 27.9055) (-11.6348, 27.9144) (-11.6419, 27.9233) (-11.6491, 27.9322) (-11.6563, 27.9411) (-11.6635, 27.95) (-11.6708, 27.9589) (-11.6781, 27.9679) (-11.6855, 27.9769) (-11.6929, 27.9859) (-11.7003, 27.9949) (-11.7078, 28.0039) (-11.7153, 28.013) (-11.7228, 28.0221) (-11.7303, 28.0312) (-11.7379, 28.0403) (-11.7456, 28.0494) (-11.7532, 28.0585) (-11.7609, 28.0677) (-11.7687, 28.0769) (-11.7765, 28.0861) (-11.7843, 28.0953) (-11.7921, 28.1045) (-11.8, 28.1137) (-11.8079, 28.123) (-11.8158, 28.1323) (-11.8238, 28.1416) (-11.8318, 28.1509) (-11.8399, 28.1602) (-11.848, 28.1695) (-11.8561, 28.1789) (-11.8643, 28.1882) (-11.8724, 28.1976) (-11.8807, 28.207) (-11.8889, 28.2164) (-11.8972, 28.2259) (-11.9055, 28.2353) (-11.9139, 28.2447) (-11.9223, 28.2542) (-11.9307, 28.2637) (-11.9392, 28.2732) (-11.9477, 28.2827) (-11.9562, 28.2922) (-11.9648, 28.3018) (-11.9734, 28.3113) (-11.982, 28.3209) (-11.9907, 28.3305) (-11.9994, 28.34) (-12.0081, 28.3496) (-12.0169, 28.3593) (-12.0257, 28.3689) (-12.0345, 28.3785) (-12.0434, 28.3882) (-12.0523, 28.3978) (-12.0613, 28.4075) (-12.0702, 28.4172) (-12.0792, 28.4269) (-12.0883, 28.4366) (-12.0973, 28.4464) (-12.1065, 28.4561) (-12.1156, 28.4658) (-12.1248, 28.4756) (-12.134, 28.4854) (-12.1432, 28.4951) (-12.1506, 28.503) (-12.1562, 28.5089) (-12.16, 28.5128) (-12.1618, 28.5147) knots 0 0 0 0 0 0 0.00416667 0.00833333 0.0125 0.01666667 0.02083333 0.025 0.02916667 0.03333333 0.0375 0.04166667 0.04583333 0.05 0.05416667 0.05833333 0.0625 0.06666667 0.07083333 0.075 0.07916667 0.08333333 0.0875 0.09166667 0.09583333 0.1 0.10416667 0.10833333 0.1125 0.11666667 0.12083333 0.125 0.12916667 0.13333333 0.1375 0.14166667 0.14583333 0.15 0.15416667 0.15833333 0.1625 0.16666667 0.17083333 0.175 0.17916667 0.18333333 0.1875 0.19166667 0.19583333 0.2 0.20416667 0.20833333 0.2125 0.21666667 0.22083333 0.225 0.22916667 0.23333333 0.2375 0.24166667 0.24583333 0.25 0.25416667 0.25833333 0.2625 0.26666667 0.27083333 0.275 0.27916667 0.28333333 0.2875 0.29166667 0.29583333 0.3 0.30416667 0.30833333 0.3125 0.31666667 0.32083333 0.325 0.32916667 0.33333333 0.3375 0.34166667 0.34583333 0.35 0.35416667 0.35833333 0.3625 0.36666667 0.37083333 0.375 0.37916667 0.38333333 0.3875 0.39166667 0.39583333 0.4 0.40416667 0.40833333 0.4125 0.41666667 0.42083333 0.425 0.42916667 0.43333333 0.4375 0.44166667 0.44583333 0.45 0.45416667 0.45833333 0.4625 0.46666667 0.47083333 0.475 0.47916667 0.48333333 0.4875 0.49166667 0.49583333 0.5 0.50416667 0.50833333 0.5125 0.51666667 0.52083333 0.525 0.52916667 0.53333333 0.5375 0.54166667 0.54583333 0.55 0.55416667 0.55833333 0.5625 0.56666667 0.57083333 0.575 0.57916667 0.58333333 0.5875 0.59166667 0.59583333 0.6 0.60416667 0.60833333 0.6125 0.61666667 0.62083333 0.625 0.62916667 0.63333333 0.6375 0.64166667 0.64583333 0.65 0.65416667 0.65833333 0.6625 0.66666667 0.67083333 0.675 0.67916667 0.68333333 0.6875 0.69166667 0.69583333 0.7 0.70416667 0.70833333 0.7125 0.71666667 0.72083333 0.725 0.72916667 0.73333333 0.7375 0.74166667 0.74583333 0.75 0.75416667 0.75833333 0.7625 0.76666667 0.77083333 0.775 0.77916667 0.78333333 0.7875 0.79166667 0.79583333 0.8 0.80416667 0.80833333 0.8125 0.81666667 0.82083333 0.825 0.82916667 0.83333333 0.8375 0.84166667 0.84583333 0.85 0.85416667 0.85833333 0.8625 0.86666667 0.87083333 0.875 0.87916667 0.88333333 0.8875 0.89166667 0.89583333 0.9 0.90416667 0.90833333 0.9125 0.91666667 0.92083333 0.925 0.92916667 0.93333333 0.9375 0.94166667 0.94583333 0.95 0.95416667 0.95833333 0.9625 0.96666667 0.97083333 0.975 0.97916667 0.98333333 0.9875 0.99166667 0.99583333 1 1 1 1 1 1
  arc A82 (-9.7471, 27.0473) -> (-10.8547, 26.6221) centre (0, 0) ccw
  spline S82 degree 5 poles (-13.0527, 28.1181) (-13.0525, 28.1154) (-13.0521, 28.11) (-13.0515, 28.1019) (-13.0506, 28.0911) (-13.0495, 28.0777) (-13.0484, 28.0644) (-13.0473, 28.051) (-13.0462, 28.0377) (-13.0451, 28.0244) (-13.0439, 28.0112) (-13.0427, 27.9979) (-13.0415, 27.9848) (-13.0404, 27.9716) (-13.0391, 27.9585) (-13.0379, 27.9454) (-13.0367, 27.9323) (-13.0354, 27.9193) (-13.0342, 27.9063) (-13.0329, 27.8934) (-13.0316, 27.8805) (-13.0303, 27.8676) (-13.029, 27.8547) (-13.0276, 27.8419) (-13.0263, 27.8291) (-13.0249, 27.8164) (-13.0236, 27.8037) (-13.0222, 27.791) (-13.0208, 27.7784) (-13.0194, 27.7658) (-13.018, 27.7532) (-13.0165, 27.7406) (-13.0151, 27.7281) (-13.0136, 27.7157) (-13.0122, 27.7032) (-13.0107, 27.6908) (-13.0092, 27.6785) (-13.0077, 27.6661) (-13.0062, 27.6539) (-13.0047, 27.6416) (-13.0031, 27.6294) (-13.0016, 27.6172) (-13, 27.605) (-12.9984, 27.5929) (-12.9968, 27.5809) (-12.9952, 27.5688) (-12.9936, 27.5568) (-12.992, 27.5449) (-12.9904, 27.5329) (-12.9887, 27.521) (-12.9871, 27.5092) (-12.9854, 27.4974) (-12.9838, 27.4856) (-12.9821, 27.4738) (-12.9804, 27.4621) (-12.9787, 27.4505) (-12.977, 27.4388) (-12.9752, 27.4273) (-12.9735, 27.4157) (-12.9718, 27.4042) (-12.97, 27.3927) (-12.9682, 27.3813) (-12.9665, 27.3699) (-12.9647, 27.3585) (-12.9629, 27.3472) (-12.9611, 27.3359) (-12.9593, 27.3247) (-12.9574, 27.3135) (-12.9556, 27.3023) (-12.9538, 27.2912) (-12.9519, 27.2801) (-12.9501, 27.2691) (-12.9482, 27.2581) (-12.9463, 27.2471) (-12.9445, 27.2362) (-12.9426, 27.2253) (-12.9407, 27.2145) (-12.9388, 27.2037) (-12.9368, 27.1929) (-12.9349, 27.1822) (-12.933, 27.1715) (-12.9311, 27.1609) (-12.9291, 27.1503) (-12.9272, 27.1397) (-12.9252, 27.1292) (-12.9232, 27.1188) (-12.9213, 27.1083) (-12.9193, 27.0979) (-12.9173, 27.0876) (-12.9153, 27.0773) (-12.9133, 27.0671) (-12.9113, 27.0568) (-12.9093, 27.0467) (-12.9072, 27.0365) (-12.9052, 27.0265) (-12.9032, 27.0164) (-12.9011, 27.0064) (-12.8991, 26.9965) (-12.8971, 26.9866) (-12.895, 26.9767) (-12.8929, 26.9669) (-12.8909, 26.9571) (-12.8888, 26.9474) (-12.8867, 26.9377) (-12.8847, 26.9281) (-12.8826, 26.9185) (-12.8805, 26.9089) (-12.8784, 26.8994) (-12.8763, 26.89) (-12.8742, 26.8806) (-12.8721, 26.8712) (-12.87, 26.8619) (-12.8679, 26.8526) (-12.8658, 26.8434) (-12.8636, 26.8342) (-12.8615, 26.8251) (-12.8594, 26.816) (-12.8573, 26.8069) (-12.8551, 26.798) (-12.853, 26.789) (-12.8509, 26.7801) (-12.8487, 26.7713) (-12.8466, 26.7625) (-12.8445, 26.7537) (-12.8423, 26.7451) (-12.8402, 26.7364) (-12.838, 26.7278) (-12.8359, 26.7193) (-12.8337, 26.7108) (-12.8316, 26.7023) (-12.8294, 26.6939) (-12.8273, 26.6856) (-12.8251, 26.6773) (-12.823, 26.669) (-12.8208, 26.6608) (-12.8187, 26.6527) (-12.8166, 26.6446) (-12.8144, 26.6365) (-12.8123, 26.6286) (-12.8101, 26.6206) (-12.808, 26.6127) (-12.8058, 26.6049) (-12.8037, 26.5971) (-12.8016, 26.5894) (-12.7994, 26.5817) (-12.7973, 26.5741) (-12.7952, 26.5665) (-12.793, 26.559) (-12.7909, 26.5516) (-12.7888, 26.5442) (-12.7867, 26.5368) (-12.7845, 26.5296) (-12.7824, 26.5223) (-12.7803, 26.5151) (-12.7782, 26.508) (-12.7761, 26.5009) (-12.774, 26.4939) (-12.772, 26.487) (-12.7699, 26.4801) (-12.7678, 26.4733) (-12.7657, 26.4665) (-12.7637, 26.4598) (-12.7616, 26.4531) (-12.7596, 26.4465) (-12.7575, 26.4399) (-12.7555, 26.4335) (-12.7534, 26.427) (-12.7514, 26.4207) (-12.7494, 26.4144) (-12.7474, 26.4081) (-12.7454, 26.4019) (-12.7434, 26.3958) (-12.7414, 26.3897) (-12.7395, 26.3837) (-12.7375, 26.3778) (-12.7356, 26.3719) (-12.7336, 26.3661) (-12.7317, 26.3604) (-12.7298, 26.3547) (-12.7279, 26.3491) (-12.726, 26.3435) (-12.7241, 26.338) (-12.7222, 26.3326) (-12.7204, 26.3273) (-12.7185, 26.322) (-12.7167, 26.3167) (-12.7149, 26.3116) (-12.7131, 26.3065) (-12.7113, 26.3015) (-12.7095, 26.2965) (-12.7077, 26.2916) (-12.706, 26.2868) (-12.7043, 26.282) (-12.7026, 26.2774) (-12.7009, 26.2728) (-12.6992, 26.2682) (-12.6975, 26.2638) (-12.6959, 26.2594) (-12.6943, 26.255) (-12.6927, 26.2508) (-12.6911, 26.2466) (-12.6895, 26.2425) (-12.688, 26.2385) (-12.6864, 26.2345) (-12.6849, 26.2307) (-12.6834, 26.2269) (-12.682, 26.2231) (-12.6806, 26.2195) (-12.6791, 26.2159) (-12.6778, 26.2124) (-12.6764, 26.209) (-12.675, 26.2057) (-12.6737, 26.2024) (-12.6724, 26.1993) (-12.6712, 26.1962) (-12.6699, 26.1932) (-12.6687, 26.1903) (-12.6676, 26.1874) (-12.6664, 26.1847) (-12.6653, 26.182) (-12.6642, 26.1794) (-12.6631, 26.1769) (-12.6621, 26.1745) (-12.6611, 26.1722) (-12.6602, 26.17) (-12.6592, 26.1678) (-12.6583, 26.1658) (-12.6575, 26.1638) (-12.6567, 26.1619) (-12.6559, 26.1602) (-12.6551, 26.1585) (-12.6544, 26.1569) (-12.6538, 26.1554) (-12.6531, 26.154) (-12.6526, 26.1527) (-12.652, 26.1515) (-12.6515, 26.1504) (-12.651, 26.1495) (-12.6506, 26.1486) (-12.6503, 26.1478) (-12.65, 26.1471) (-12.6497, 26.1467) (-12.6496, 26.1464) (-12.6495, 26.1462) (-12.6495, 26.1461) knots -1 -1 -1 -1 -1 -1 -0.99583333 -0.99166667 -0.9875 -0.98333333 -0.97916667 -0.975 -0.97083333 -0.96666667 -0.9625 -0.95833333 -0.95416667 -0.95 -0.94583333 -0.94166667 -0.9375 -0.93333333 -0.92916667 -0.925 -0.92083333 -0.91666667 -0.9125 -0.90833333 -0.90416667 -0.9 -0.89583333 -0.89166667 -0.8875 -0.88333333 -0.87916667 -0.875 -0.87083333 -0.86666667 -0.8625 -0.85833333 -0.85416667 -0.85 -0.84583333 -0.84166667 -0.8375 -0.83333333 -0.82916667 -0.825 -0.82083333 -0.81666667 -0.8125 -0.80833333 -0.80416667 -0.8 -0.79583333 -0.79166667 -0.7875 -0.78333333 -0.77916667 -0.775 -0.77083333 -0.76666667 -0.7625 -0.75833333 -0.75416667 -0.75 -0.74583333 -0.74166667 -0.7375 -0.73333333 -0.72916667 -0.725 -0.72083333 -0.71666667 -0.7125 -0.70833333 -0.70416667 -0.7 -0.69583333 -0.69166667 -0.6875 -0.68333333 -0.67916667 -0.675 -0.67083333 -0.66666667 -0.6625 -0.65833333 -0.65416667 -0.65 -0.64583333 -0.64166667 -0.6375 -0.63333333 -0.62916667 -0.625 -0.62083333 -0.61666667 -0.6125 -0.60833333 -0.60416667 -0.6 -0.59583333 -0.59166667 -0.5875 -0.58333333 -0.57916667 -0.575 -0.57083333 -0.56666667 -0.5625 -0.55833333 -0.55416667 -0.55 -0.54583333 -0.54166667 -0.5375 -0.53333333 -0.52916667 -0.525 -0.52083333 -0.51666667 -0.5125 -0.50833333 -0.50416667 -0.5 -0.49583333 -0.49166667 -0.4875 -0.48333333 -0.47916667 -0.475 -0.47083333 -0.46666667 -0.4625 -0.45833333 -0.45416667 -0.45 -0.44583333 -0.44166667 -0.4375 -0.43333333 -0.42916667 -0.425 -0.42083333 -0.41666667 -0.4125 -0.40833333 -0.40416667 -0.4 -0.39583333 -0.39166667 -0.3875 -0.38333333 -0.37916667 -0.375 -0.37083333 -0.36666667 -0.3625 -0.35833333 -0.35416667 -0.35 -0.34583333 -0.34166667 -0.3375 -0.33333333 -0.32916667 -0.325 -0.32083333 -0.31666667 -0.3125 -0.30833333 -0.30416667 -0.3 -0.29583333 -0.29166667 -0.2875 -0.28333333 -0.27916667 -0.275 -0.27083333 -0.26666667 -0.2625 -0.25833333 -0.25416667 -0.25 -0.24583333 -0.24166667 -0.2375 -0.23333333 -0.22916667 -0.225 -0.22083333 -0.21666667 -0.2125 -0.20833333 -0.20416667 -0.2 -0.19583333 -0.19166667 -0.1875 -0.18333333 -0.17916667 -0.175 -0.17083333 -0.16666667 -0.1625 -0.15833333 -0.15416667 -0.15 -0.14583333 -0.14166667 -0.1375 -0.13333333 -0.12916667 -0.125 -0.12083333 -0.11666667 -0.1125 -0.10833333 -0.10416667 -0.1 -0.09583333 -0.09166667 -0.0875 -0.08333333 -0.07916667 -0.075 -0.07083333 -0.06666667 -0.0625 -0.05833333 -0.05416667 -0.05 -0.04583333 -0.04166667 -0.0375 -0.03333333 -0.02916667 -0.025 -0.02083333 -0.01666667 -0.0125 -0.00833333 -0.00416667 0 0 0 0 0 0
  spline S83 degree 5 poles (-6.9214, 30.2174) (-6.9218, 30.2148) (-6.9225, 30.2094) (-6.9236, 30.2014) (-6.925, 30.1907) (-6.9267, 30.1773) (-6.9284, 30.164) (-6.9301, 30.1507) (-6.9317, 30.1375) (-6.9334, 30.1242) (-6.935, 30.111) (-6.9366, 30.0979) (-6.9382, 30.0847) (-6.9398, 30.0716) (-6.9413, 30.0585) (-6.9428, 30.0455) (-6.9443, 30.0324) (-6.9458, 30.0194) (-6.9473, 30.0065) (-6.9487, 29.9935) (-6.9501, 29.9806) (-6.9516, 29.9678) (-6.9529, 29.9549) (-6.9543, 29.9421) (-6.9556, 29.9293) (-6.957, 29.9166) (-6.9583, 29.9039) (-6.9596, 29.8912) (-6.9608, 29.8785) (-6.9621, 29.8659) (-6.9633, 29.8533) (-6.9645, 29.8407) (-6.9657, 29.8282) (-6.9669, 29.8157) (-6.968, 29.8032) (-6.9691, 29.7908) (-6.9702, 29.7784) (-6.9713, 29.766) (-6.9724, 29.7537) (-6.9735, 29.7414) (-6.9745, 29.7291) (-6.9755, 29.7169) (-6.9765, 29.7047) (-6.9775, 29.6925) (-6.9784, 29.6803) (-6.9794, 29.6682) (-6.9803, 29.6562) (-6.9812, 29.6441) (-6.9821, 29.6321) (-6.983, 29.6201) (-6.9838, 29.6082) (-6.9846, 29.5963) (-6.9855, 29.5844) (-6.9863, 29.5726) (-6.987, 29.5608) (-6.9878, 29.549) (-6.9885, 29.5373) (-6.9892, 29.5256) (-6.99, 29.514) (-6.9906, 29.5023) (-6.9913, 29.4907) (-6.992, 29.4792) (-6.9926, 29.4677) (-6.9932, 29.4562) (-6.9938, 29.4447) (-6.9944, 29.4333) (-6.995, 29.422) (-6.9955, 29.4106) (-6.996, 29.3993) (-6.9965, 29.3881) (-6.997, 29.3768) (-6.9975, 29.3657) (-6.998, 29.3545) (-6.9984, 29.3434) (-6.9989, 29.3323) (-6.9993, 29.3213) (-6.9997, 29.3103) (-7.0001, 29.2993) (-7.0004, 29.2884) (-7.0008, 29.2775) (-7.0011, 29.2667) (-7.0014, 29.2559) (-7.0017, 29.2451) (-7.002, 29.2344) (-7.0023, 29.2237) (-7.0025, 29.213) (-7.0028, 29.2024) (-7.003, 29.1919) (-7.0032, 29.1813) (-7.0034, 29.1708) (-7.0035, 29.1604) (-7.0037, 29.15) (-7.0038, 29.1396) (-7.004, 29.1293) (-7.0041, 29.119) (-7.0042, 29.1088) (-7.0043, 29.0986) (-7.0043, 29.0884) (-7.0044, 29.0783) (-7.0044, 29.0682) (-7.0045, 29.0582) (-7.0045, 29.0482) (-7.0045, 29.0383) (-7.0045, 29.0284) (-7.0044, 29.0185) (-7.0044, 29.0087) (-7.0043, 28.9989) (-7.0043, 28.9892) (-7.0042, 28.9795) (-7.0041, 28.9698) (-7.004, 28.9602) (-7.0038, 28.9507) (-7.0037, 28.9412) (-7.0036, 28.9317) (-7.0034, 28.9223) (-7.0032, 28.9129) (-7.003, 28.9036) (-7.0028, 28.8943) (-7.0026, 28.8851) (-7.0024, 28.8759) (-7.0021, 28.8668) (-7.0019, 28.8577) (-7.0016, 28.8486) (-7.0014, 28.8396) (-7.0011, 28.8307) (-7.0008, 28.8218) (-7.0005, 28.8129) (-7.0001, 28.8041) (-6.9998, 28.7953) (-6.9995, 28.7866) (-6.9991, 28.778) (-6.9987, 28.7694) (-6.9984, 28.7608) (-6.998, 28.7523) (-6.9976, 28.7438) (-6.9972, 28.7354) (-6.9968, 28.727) (-6.9963, 28.7187) (-6.9959, 28.7105) (-6.9954, 28.7023) (-6.995, 28.6941) (-6.9945, 28.686) (-6.994, 28.678) (-6.9936, 28.67) (-6.9931, 28.662) (-6.9926, 28.6541) (-6.9921, 28.6463) (-6.9915, 28.6385) (-6.991, 28.6307) (-6.9905, 28.6231) (-6.9899, 28.6154) (-6.9894, 28.6079) (-6.9888, 28.6004) (-6.9882, 28.5929) (-6.9877, 28.5855) (-6.9871, 28.5781) (-6.9865, 28.5709) (-6.9859, 28.5636) (-6.9853, 28.5564) (-6.9847, 28.5493) (-6.9841, 28.5423) (-6.9835, 28.5353) (-6.9828, 28.5283) (-6.9822, 28.5214) (-6.9816, 28.5146) (-6.9809, 28.5078) (-6.9803, 28.5011) (-6.9796, 28.4945) (-6.9789, 28.4879) (-6.9783, 28.4814) (-6.9776, 28.4749) (-6.9769, 28.4685) (-6.9763, 28.4622) (-6.9756, 28.4559) (-6.9749, 28.4497) (-6.9742, 28.4435) (-6.9735, 28.4374) (-6.9728, 28.4314) (-6.9721, 28.4255) (-6.9714, 28.4196) (-6.9707, 28.4137) (-6.97, 28.408) (-6.9693, 28.4023) (-6.9686, 28.3966) (-6.9679, 28.3911) (-6.9672, 28.3856) (-6.9665, 28.3802) (-6.9658, 28.3748) (-6.9651, 28.3695) (-6.9644, 28.3643) (-6.9637, 28.3592) (-6.963, 28.3541) (-6.9623, 28.3491) (-6.9616, 28.3442) (-6.9609, 28.3393) (-6.9602, 28.3345) (-6.9595, 28.3298) (-6.9588, 28.3252) (-6.9581, 28.3206) (-6.9574, 28.3161) (-6.9568, 28.3117) (-6.9561, 28.3074) (-6.9554, 28.3031) (-6.9547, 28.2989) (-6.9541, 28.2948) (-6.9534, 28.2908) (-6.9528, 28.2868) (-6.9521, 28.283) (-6.9515, 28.2792) (-6.9508, 28.2755) (-6.9502, 28.2719) (-6.9496, 28.2683) (-6.949, 28.2649) (-6.9484, 28.2615) (-6.9478, 28.2582) (-6.9472, 28.255) (-6.9466, 28.2519) (-6.9461, 28.2489) (-6.9455, 28.246) (-6.945, 28.2431) (-6.9445, 28.2404) (-6.9439, 28.2377) (-6.9434, 28.2351) (-6.9429, 28.2327) (-6.9425, 28.2303) (-6.942, 28.228) (-6.9416, 28.2258) (-6.9411, 28.2237) (-6.9407, 28.2217) (-6.9403, 28.2198) (-6.9399, 28.218) (-6.9396, 28.2163) (-6.9392, 28.2147) (-6.9389, 28.2132) (-6.9386, 28.2118) (-6.9383, 28.2106) (-6.9381, 28.2094) (-6.9378, 28.2083) (-6.9376, 28.2074) (-6.9374, 28.2065) (-6.9372, 28.2058) (-6.9371, 28.2053) (-6.937, 28.205) (-6.937, 28.2048) (-6.937, 28.2047) knots -1 -1 -1 -1 -1 -1 -0.99583333 -0.99166667 -0.9875 -0.98333333 -0.97916667 -0.975 -0.97083333 -0.96666667 -0.9625 -0.95833333 -0.95416667 -0.95 -0.94583333 -0.94166667 -0.9375 -0.93333333 -0.92916667 -0.925 -0.92083333 -0.91666667 -0.9125 -0.90833333 -0.90416667 -0.9 -0.89583333 -0.89166667 -0.8875 -0.88333333 -0.87916667 -0.875 -0.87083333 -0.86666667 -0.8625 -0.85833333 -0.85416667 -0.85 -0.84583333 -0.84166667 -0.8375 -0.83333333 -0.82916667 -0.825 -0.82083333 -0.81666667 -0.8125 -0.80833333 -0.80416667 -0.8 -0.79583333 -0.79166667 -0.7875 -0.78333333 -0.77916667 -0.775 -0.77083333 -0.76666667 -0.7625 -0.75833333 -0.75416667 -0.75 -0.74583333 -0.74166667 -0.7375 -0.73333333 -0.72916667 -0.725 -0.72083333 -0.71666667 -0.7125 -0.70833333 -0.70416667 -0.7 -0.69583333 -0.69166667 -0.6875 -0.68333333 -0.67916667 -0.675 -0.67083333 -0.66666667 -0.6625 -0.65833333 -0.65416667 -0.65 -0.64583333 -0.64166667 -0.6375 -0.63333333 -0.62916667 -0.625 -0.62083333 -0.61666667 -0.6125 -0.60833333 -0.60416667 -0.6 -0.59583333 -0.59166667 -0.5875 -0.58333333 -0.57916667 -0.575 -0.57083333 -0.56666667 -0.5625 -0.55833333 -0.55416667 -0.55 -0.54583333 -0.54166667 -0.5375 -0.53333333 -0.52916667 -0.525 -0.52083333 -0.51666667 -0.5125 -0.50833333 -0.50416667 -0.5 -0.49583333 -0.49166667 -0.4875 -0.48333333 -0.47916667 -0.475 -0.47083333 -0.46666667 -0.4625 -0.45833333 -0.45416667 -0.45 -0.44583333 -0.44166667 -0.4375 -0.43333333 -0.42916667 -0.425 -0.42083333 -0.41666667 -0.4125 -0.40833333 -0.40416667 -0.4 -0.39583333 -0.39166667 -0.3875 -0.38333333 -0.37916667 -0.375 -0.37083333 -0.36666667 -0.3625 -0.35833333 -0.35416667 -0.35 -0.34583333 -0.34166667 -0.3375 -0.33333333 -0.32916667 -0.325 -0.32083333 -0.31666667 -0.3125 -0.30833333 -0.30416667 -0.3 -0.29583333 -0.29166667 -0.2875 -0.28333333 -0.27916667 -0.275 -0.27083333 -0.26666667 -0.2625 -0.25833333 -0.25416667 -0.25 -0.24583333 -0.24166667 -0.2375 -0.23333333 -0.22916667 -0.225 -0.22083333 -0.21666667 -0.2125 -0.20833333 -0.20416667 -0.2 -0.19583333 -0.19166667 -0.1875 -0.18333333 -0.17916667 -0.175 -0.17083333 -0.16666667 -0.1625 -0.15833333 -0.15416667 -0.15 -0.14583333 -0.14166667 -0.1375 -0.13333333 -0.12916667 -0.125 -0.12083333 -0.11666667 -0.1125 -0.10833333 -0.10416667 -0.1 -0.09583333 -0.09166667 -0.0875 -0.08333333 -0.07916667 -0.075 -0.07083333 -0.06666667 -0.0625 -0.05833333 -0.05416667 -0.05 -0.04583333 -0.04166667 -0.0375 -0.03333333 -0.02916667 -0.025 -0.02083333 -0.01666667 -0.0125 -0.00833333 -0.00416667 0 0 0 0 0 0
  line L171 (-6.9368, -28.2039) -> (-6.937, -28.2047)
  line L172 (-8.0945, 27.8937) -> (-8.0948, 27.8945)
  line L173 (10.9659, 26.8948) -> (10.8547, 26.6221)
  line L174 (9.8469, 27.3243) -> (9.8472, 27.3251)
  line L175 (-28.7355, 0.9119) -> (-29.0298, 0.9213)
  line L176 (-29.0298, 0.9213) -> (-29.0307, 0.9213)
  line L177 (9.7471, 27.0473) -> (9.8469, 27.3243)
  line L178 (-8.0125, 27.6109) -> (-8.0945, 27.8937)
  line L179 (10.9662, 26.8955) -> (10.9659, 26.8948)